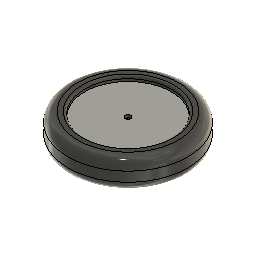
Roue (Autodesk Fusion 360 design; units mm, degrees)
Autodesk Fusion 360 part; units mm, degrees
sketch "Sketch1" plane through (0, 0, 0) normal (0, 0, 1) x (1, 0, 0)
  circle A0 centre (0, 0) radius 62
  circle A1 centre (0, 0) radius 45
  circle A2 centre (0, 0) radius 3
  dimension "d1" = 124
  dimension "d5" = 90
  dimension "d14" = 6
  constraint coincident A0.centre A1.centre
  measures "d1" diameter of A0 A1.centre
  measures "d5" diameter of A1
  measures "d14" diameter of A2
extrude "Extrude1" add sketch "Sketch1" along normal blind 30 contours A0 | A1 | A2
fillet "Fillet1" radius 10 2 edges at (-57.8043, -22.4202, 30) (-57.8043, -22.4202, 0)
sketch "Sketch4" plane through (0, 0, 0) normal (0, 0, -1) x (1, 0, 0)
  circle A0 centre (0, 0) radius 52
  line L0 (6.9152, -1.8529) -> (5.0623, 5.0623)
  line L1 (5.0623, 5.0623) -> (-1.8529, 6.9152)
  line L2 (-1.8529, 6.9152) -> (-6.9152, 1.8529)
  line L3 (-6.9152, 1.8529) -> (-5.0623, -5.0623)
  line L4 (-5.0623, -5.0623) -> (1.8529, -6.9152)
  line L5 (1.8529, -6.9152) -> (6.9152, -1.8529)
  dimension "d16" = 12.4
  constraint coincident A0.centre origin
  measures "d16" distance of L2 L5
extrude "Extrude5" cut sketch "Sketch4" against normal blind 22 contours L0 L1 L2 L3 L4 L5
extrude "Extrude2" cut sketch "Sketch1" along normal blind 5 contours A1 | A2
sketch "Sketch3" plane through (0, 0, 30) normal (0, 0, 1) x (-1, 0, 0)
  circle A0 centre (0, 0) radius 52
  circle A1 centre (0, 0) radius 45
  dimension "d9" = 90
  constraint coincident A0.centre A1.centre
  measures "d9" diameter of A1
extrude "Extrude3" cut sketch "Sketch3" against normal blind 5 contours A1
fillet "Fillet2" radius 2.5 1 edges at (41.9547, -16.2727, 30)
fillet "Fillet3" radius 2.5 1 edges at (-41.9547, -16.2727, 0)
extrude "Extrude4" cut sketch "Sketch1" along normal through all contours A2
